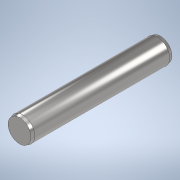
# Autodesk Inventor part: 平行ピンD4L23
Saved by Autodesk Inventor 2020.2 (Build 242310000, 310)
## iProperties
Created: 2020-02-29
Part Number: 平行ピンD4L23
Material: ステンレス鋼
Document SubType Name: Modeling
Designer: aoyam
Density: 8 g/cm^3
Appearance: 半つや出し
Author: aoyam
Autodesk Inventor part; units mm, degrees
ref_plane "YZ Plane" through (0, 0, 0) normal (1, 0, 0) x (0, 1, 0)
ref_plane "XZ Plane" through (0, 0, 0) normal (0, 1, 0) x (-1, 0, 0)
ref_plane "XY Plane" through (0, 0, 0) normal (0, 0, 1) x (1, 0, 0)
sketch "スケッチ1" plane through (0, 0, 0) normal (0, 0, 1) x (1, 0, 0)
  circle A0 centre (0, 0) radius 2
  dimension "d0" = 4
  constraints: 1 centre point, 1 coincident
  measures "d0" diameter of A0
extrude "押し出し1" add sketch "スケッチ1" along normal blind 23
chamfer "面取り1" distance 0.5 angle 15 2 edges at (-2, 0, 0) (-2, 0, 23) measured on face at (1.9741, -0.3208, 15.3333)
